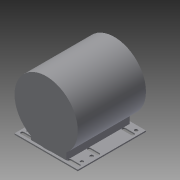
# Autodesk Inventor part: Motor5
Saved by Autodesk Inventor 2015 SP1 (Build 190203100, 203)
## iProperties
Created: 2016-02-24
Part Number: Motor5
Material: Generic
Document SubType Name: Modeling
Designer: jonesdm
Density: 1 g/cm^3
Appearance: Default
Author: jonesdm
Autodesk Inventor part; units mm, degrees
ref_plane "YZ Plane" through (0, 0, 0) normal (1, 0, 0) x (0, 1, 0)
ref_plane "XZ Plane" through (0, 0, 0) normal (0, 1, 0) x (-1, 0, 0)
ref_plane "XY Plane" through (0, 0, 0) normal (0, 0, 1) x (1, 0, 0)
sketch "Sketch1" plane through (0, 0, 0) normal (0, 0, 1) x (1, 0, 0)
  circle A0 centre (0, 0) radius 7.9375
  line L0 (-2.4257, 7.5578) -> (-2.4257, 10.0978)
  line L1 (-2.4257, 10.0978) -> (2.4257, 10.0978)
  line L2 (2.4257, 10.0978) -> (2.4257, 7.5578)
  point P0 (0, 10.0978)
  dimension "d0" = 15.875
  dimension "d1" = 2.54
  dimension "d2" = 4.8514
  constraints: 6 end point, 2 point on circle, 1 centre point, 1 coincident, 1 horizontal, 1 midpoint, 1 perpendicular, 1 vertical, 1 vertical alignment
  measures "d0" diameter of A0
  measures "d1" distance of L1.end L2.end
  measures "d2" distance of L0.end L1.end
extrude "Extrusion1" add sketch "Sketch1" along normal blind 50.8
sketch "Sketch2" plane through (0, 0, 50.8) normal (0, 0, 1) x (1, 0, 0)
  circle A0 centre (0, 0) radius 82.55
  dimension "d5" = 165.1
  constraints: 1 centre point, 1 coincident
  measures "d5" diameter of A0
extrude "Extrusion2" add sketch "Sketch2" along normal blind 177.8
sketch "Sketch3" plane through (0, 0, 50.8) normal (0, 0, -1) x (-1, 0, 0)
  circle A0 centre (0, 0) radius 73.025
  arc A1 (-2.4257, 7.5578) -> (2.4257, 7.5578) centre (0, 0) ccw projected
  line L0 (0, 0) -> (51.6365, 51.6365)
  line L1 (0, 0) -> (73.025, 0) construction
  line L2 (0, 0) -> (51.6365, -51.6365)
  line L3 (0, 0) -> (73.025, 0) construction
  line L4 (0, 0) -> (-51.6365, 51.6365)
  line L5 (0, 0) -> (73.025, 0) construction
  line L6 (0, 0) -> (-51.6365, -51.6365)
  line L7 (0, 0) -> (73.025, 0) construction
  dimension "d8" = 146.05
  dimension "d9" = 45
  dimension "d10" = 45
  dimension "d11" = 135
  dimension "d12" = 135
  constraints: 16 end point, 5 coincident, 4 equal length, 4 horizontal, 4 point on circle, 1 centre point
  measures "d8" diameter of A0
  measures "d9" angle of L1 L0
  measures "d10" angle of L2 L3
  measures "d11" angle of L5 L4
  measures "d12" angle of L6 L7
hole "Hole1" at (51.6365, 51.6365, 50.8) at (-51.6365, 51.6365, 50.8) at (-51.6365, -51.6365, 50.8) at (51.6365, -51.6365, 50.8) direction (0, 0, 1) diameter 4.9784 depth 19.05 tip angle 118 thread size "1/4-20 UNC" class "2B" standard "ANSI Unified Screw Threads"
ref_plane "Work Plane2" through (0, -82.55, 50.8) normal (0, 1, 0) x (-1, 0, 0)
sketch "Sketch4" plane through (0, -82.55, 50.8) normal (0, 1, 0) x (-1, 0, 0)
  line L0 (82.55, 177.8) -> (-82.55, 177.8) projected
  line L1 (-82.55, 0) -> (82.55, 0) projected
  line L2 (82.55, 0) -> (82.55, 177.8) projected
  line L3 (-82.55, 0) -> (-82.55, 177.8) projected
  line L4 (-46.355, 6.35) -> (46.355, 6.35)
  line L5 (46.355, 6.35) -> (46.355, 171.45)
  line L6 (46.355, 171.45) -> (-46.355, 171.45)
  line L7 (-46.355, 171.45) -> (-46.355, 6.35)
  point P0 (0, -50.8)
  point P1 (0, 6.35)
  dimension "d20" = 165.1
  dimension "d21" = 6.35
  dimension "d22" = 92.71
  constraints: 8 end point, 2 parallel, 1 horizontal, 1 midpoint, 1 perpendicular, 1 vertical alignment
  measures "d20" distance of L4.end L5.end
  measures "d21" distance between parallel lines of L1 L4
  measures "d22" distance of L4.start L4.end
extrude "Extrusion3" add sketch "Sketch4" along normal blind 25.4 and the other way blind 5.2324 contours L7 L6 L5 L4
ref_plane "Work Plane7" through (0, -90.9574, 50.8) normal (0, -1, 0) x (1, 0, 0)
sketch "Sketch5" plane through (0, -90.9574, 50.8) normal (0, -1, 0) x (1, 0, 0)
  line L0 (82.55, 177.8) -> (-82.55, 177.8) projected
  line L1 (-82.55, 0) -> (82.55, 0) projected
  line L2 (82.4515, 177.8) -> (-82.55, 177.8)
  line L3 (-82.55, 177.8) -> (-82.55, 0)
  line L4 (-82.55, 0) -> (82.4515, 0)
  line L5 (82.4515, 0) -> (82.4515, 177.8)
  point P0 (0, -50.8)
  constraints: 9 end point, 2 parallel, 1 horizontal, 1 perpendicular, 1 point on line
extrude "Extrusion4" add sketch "Sketch5" against normal blind 3.175
ref_plane "Work Plane9" through (0, -94.1324, 50.8) normal (0, -1, 0) x (1, 0, 0)
sketch "Sketch6" plane through (0, -94.1324, 50.8) normal (0, -1, 0) x (1, 0, 0)
  circle A0 centre (69.4594, 154.0383) radius 4.2291
  line L0 (82.4515, 0) -> (82.4515, 177.8) projected
  line L1 (82.4515, 177.8) -> (-82.55, 177.8) projected
  line L2 (73.1424, 171.0436) -> (50.2316, 171.0436)
  line L3 (50.2316, 162.5854) -> (73.1424, 162.5854)
  line L4 (77.3259, 166.1953) -> (77.3259, 167.4337)
  arc A1 (73.1424, 162.5854) -> (73.1424, 171.0436) centre (73.1424, 166.8145) ccw
  arc A2 (50.2316, 171.0436) -> (50.2316, 162.5854) centre (50.2316, 166.8145) ccw
  line L5 (82.55, 177.8) -> (-82.55, 177.8) projected
  line L6 (-2.4257, -50.8) -> (-2.4257, 0) projected
  circle A3 centre (69.4594, 128.7145) radius 4.2291
  line L7 (73.1424, 111.7092) -> (50.2316, 111.7092)
  line L8 (50.2316, 120.1674) -> (73.1424, 120.1674)
  arc A4 (73.1424, 111.7092) -> (73.1424, 120.1674) centre (73.1424, 115.9383) ccw
  arc A5 (50.2316, 120.1674) -> (50.2316, 111.7092) centre (50.2316, 115.9383) ccw
  arc A6 (73.1424, 21.1836) -> (73.1424, 29.6418) centre (73.1424, 25.4127) ccw
  line L9 (50.2316, 21.1836) -> (73.1424, 21.1836)
  line L10 (73.1424, 29.6418) -> (50.2316, 29.6418)
  arc A7 (50.2316, 29.6418) -> (50.2316, 21.1836) centre (50.2316, 25.4127) ccw
  circle A8 centre (69.4594, 12.6365) radius 4.2291
  line L11 (-82.55, 0) -> (82.4515, 0) projected
  circle A9 centre (-69.4594, 154.0383) radius 4.2291
  line L12 (-73.1424, 171.0436) -> (-50.2316, 171.0436)
  line L13 (-50.2316, 162.5854) -> (-73.1424, 162.5854)
  line L14 (-77.3259, 166.1953) -> (-77.3259, 167.4337)
  arc A10 (-73.1424, 171.0436) -> (-73.1424, 162.5854) centre (-73.1424, 166.8145) ccw
  arc A11 (-50.2316, 162.5854) -> (-50.2316, 171.0436) centre (-50.2316, 166.8145) ccw
  arc A12 (-73.1424, 120.1674) -> (-73.1424, 111.7092) centre (-73.1424, 115.9383) ccw
  line L15 (-50.2316, 120.1674) -> (-73.1424, 120.1674)
  line L16 (-73.1424, 111.7092) -> (-50.2316, 111.7092)
  arc A13 (-50.2316, 111.7092) -> (-50.2316, 120.1674) centre (-50.2316, 115.9383) ccw
  circle A14 centre (-69.4594, 128.7145) radius 4.2291
  circle A15 centre (-69.4594, 12.6365) radius 4.2291
  line L17 (-50.2316, 21.1836) -> (-73.1424, 21.1836)
  line L18 (-73.1424, 29.6418) -> (-50.2316, 29.6418)
  arc A16 (-73.1424, 29.6418) -> (-73.1424, 21.1836) centre (-73.1424, 25.4127) ccw
  arc A17 (-50.2316, 21.1836) -> (-50.2316, 29.6418) centre (-50.2316, 25.4127) ccw
  point P0 (0, -50.8)
  dimension "d31" = 8.4582
  dimension "d32" = 12.9921
  dimension "d33" = 23.7617
  dimension "d38" = 8.4582
  dimension "d39" = 8.4582
  dimension "d40" = 22.9108
  dimension "d41" = 8.4582
  dimension "d46" = 6.7564
  dimension "d47" = 9.3091
  dimension "d50" = 12.6365
  dimension "d51" = 8.5471
  constraints: 28 end point, 28 point on circle, 18 centre point, 1 horizontal, 1 parallel
  measures "d31" diameter of A0
  measures "d32" distance from line of L0 A0.centre
  measures "d33" distance from line of A0.centre L1
  measures "d38" diameter of A1
  measures "d39" diameter of A2
  measures "d40" distance of A2.centre A1.centre
  measures "d41" distance between parallel lines of L3 L2
  measures "d46" distance between parallel lines of L2 L1
  measures "d47" distance from line of L0 A1.centre
  measures "d50" distance from line of A8.centre L11
  measures "d51" distance from line of L9 A8.centre
extrude "Extrusion5" cut sketch "Sketch6" against normal blind 6.35 contours A0 | A1 L4 L3 A2 L2 | A3 | L7 A5 L8 A4 | L9 A7 L10 A6 | A8 | A9 | L12 A11 L13 A10 L14 | L15 A13 L16 A12 | A14 | A15 | L17 A16 L18 A17
sketch "Sketch7" plane through (0, -87.7824, 50.8) normal (0, -1, 0) x (1, 0, 0)
  point P0 (0, -50.8)
equation "\"d3\" = ShaftL"
equation "\"d5\" = MotoD"
equation "\"d6\" = MotoL"
equation "\"ShaftL\" = 50.8"
equation "\"MotoD\" = 165.1"
equation "\"MotoL\" = 177.8"
body "Solid1"
